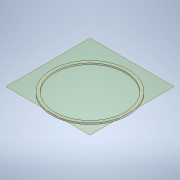
# Autodesk Inventor part: UpperSailCapBottom-ver1-1111-2021
Saved by Autodesk Inventor 2021 (Build 250183000, 183)
## iProperties
Created: 2021-01-28
Part Number: UpperSailCapBottom-ver1-1111-2021
Material: Generic
Document SubType Name: Modeling
Designer: con_c_000
Density: 1 g/cm^3
Appearance: Default
Author: con_c_000
Autodesk Inventor part; units mm, degrees
sketch "Sketch1" plane through (0, 0, 0) normal (0, 1, 0) x (-1, 0, 0)
  circle A0 centre (0, 0) radius 152.4
  circle A1 centre (0, 0) radius 165.1
  dimension "d0" = 304.8
  dimension "d1" = 330.2
  constraints: 2 centre point, 2 coincident
  measures "d0" diameter of A0
  measures "d1" diameter of A1
extrude "Extrusion1" add sketch "Sketch1" along normal blind 152.4
sketch "Sketch2" plane through (0, 0, 0) normal (1, 0, 0) x (0, 1, 0)
  circle A0 centre (100.6077, 0) radius 25.4
  point P0 (0, 0)
  dimension "d4" = 50.8
  constraints: 1 centre point
  measures "d4" diameter of A0
extrude "Extrusion2" add sketch "Sketch2" along normal mid plane 889
sketch "Sketch4" plane through (0, 152.4, 0) normal (0, 1, 0) x (1, 0, 0)
  circle A0 centre (0, 0) radius 152.4
  constraints: 1 centre point, 1 coincident
extrude "Extrusion4" cut sketch "Sketch4" against normal through all
sketch "Sketch5" plane through (0, 152.4, 0) normal (0, 1, 0) x (1, 0, 0)
  circle A0 centre (0, 0) radius 165.1
  constraints: 1 centre point, 1 coincident
extrude "Extrusion5" add sketch "Sketch5" along normal blind 50.8 draft -50
ref_plane "Work Plane2" through (75.376, -18.8821, -44.9646) normal (1, 0, 0) x (0, 1, 0)
ref_plane "Work Plane5" through (0, 25.4, 165.1) normal (0, 0, 1) x (1, 0, 0)
sketch "Sketch11" plane through (0, 25.4, 165.1) normal (0, 0, 1) x (1, 0, 0)
  circle A0 centre (0, 75.2094) radius 25.4
  line L0 (165.1, -25.4) -> (-165.1, -25.4) projected
  point P0 (0, -25.4)
  dimension "d31" = 50.8
  dimension "d32" = 100.6094
  constraints: 1 centre point
  measures "d31" diameter of A0
  measures "d32" distance from line of L0 A0.centre
extrude "Extrusion11" add sketch "Sketch11" along normal blind 280.543
ref_plane "Work Plane6" through (0, 25.4, -165.1) normal (0, 0, 1) x (1, 0, 0)
sketch "Sketch12" plane through (0, 25.4, -165.1) normal (0, 0, 1) x (1, 0, 0)
  circle A0 centre (0, 75.2094) radius 25.4
  line L0 (165.1, -25.4) -> (-165.1, -25.4) projected
  point P0 (0, -25.4)
  dimension "d36" = 50.8
  dimension "d37" = 100.6094
  constraints: 1 centre point
  measures "d36" diameter of A0
  measures "d37" distance from line of L0 A0.centre
extrude "Extrusion12" add sketch "Sketch12" against normal blind 280.543
ref_plane "Work Plane10" through (0, 152.4, 0) normal (0, -1, 0) x (1, 0, 0)
ref_plane "Work Plane9" through (0, 63.5, 0) normal (0, -1, 0) x (1, 0, 0)
sketch "Sketch13" plane through (0, 152.4, 0) normal (0, -1, 0) x (1, 0, 0)
  line L0 (-199.2875, -201.2037) -> (234.7376, -201.2037)
  line L1 (234.7376, -201.2037) -> (234.7376, 210.7848)
  line L2 (234.7376, 210.7848) -> (-199.2875, 210.7848)
  line L3 (-199.2875, 210.7848) -> (-199.2875, -201.2037)
  point P0 (0, 0)
  constraints: 8 end point, 2 parallel, 1 horizontal, 1 perpendicular
extrude "Extrusion13" cut sketch "Sketch13" against normal blind 127
ref_plane "Work Plane11" through (0, 63.5, 0) normal (0, -1, 0) x (1, 0, 0)
sketch "Sketch15" plane through (0, 63.5, 0) normal (0, -1, 0) x (1, 0, 0)
  line L0 (-509.2014, 528.9036) -> (494.7202, 528.9036)
  line L1 (494.7202, 528.9036) -> (494.7202, -498.4488)
  line L2 (494.7202, -498.4488) -> (-509.2014, -498.4488)
  line L3 (-509.2014, -498.4488) -> (-509.2014, 528.9036)
  point P0 (0, 0)
  constraints: 8 end point, 2 parallel, 1 horizontal, 1 perpendicular
extrude "Extrusion15" cut sketch "Sketch15" against normal blind 254
ref_plane "Work Plane12" through (0, 25.4, 0) normal (0, -1, 0) x (1, 0, 0)
sketch "Sketch16" plane through (0, 25.4, 0) normal (0, -1, 0) x (1, 0, 0)
  line L0 (-189.4244, 211.7722) -> (231.9916, 211.7722)
  line L1 (231.9916, 211.7722) -> (231.9916, -229.8633)
  line L2 (231.9916, -229.8633) -> (-189.4244, -229.8633)
  line L3 (-189.4244, -229.8633) -> (-189.4244, 211.7722)
  point P0 (0, 0)
  constraints: 8 end point, 2 parallel, 1 horizontal, 1 perpendicular
extrude "Extrusion16" cut sketch "Sketch16" against normal blind 254
ref_plane "Work Plane14" through (-0.824, -18.8821, -44.9646) normal (1, 0, 0) x (0, 1, 0)
ref_plane "Work Plane13" through (164.276, -18.8821, -44.9646) normal (1, 0, 0) x (0, 1, 0)
ref_plane "Work Plane15" through (0, 25.4, 0) normal (0, -1, 0) x (1, 0, 0)
sketch "Sketch17" plane through (0, 25.4, 0) normal (0, -1, 0) x (1, 0, 0)
  line L0 (-206.305, -203.3787) -> (218.0102, -203.3787)
  line L1 (218.0102, -203.3787) -> (218.0102, 226.7892)
  line L2 (218.0102, 226.7892) -> (-206.305, 226.7892)
  line L3 (-206.305, 226.7892) -> (-206.305, -203.3787)
  point P0 (0, 0)
  constraints: 8 end point, 2 parallel, 1 horizontal, 1 perpendicular
extrude "Extrusion17" cut sketch "Sketch17" along normal blind 19.05
ref_plane "Work Plane8" through (0, 0, 0) normal (0, -1, 0) x (1, 0, 0)
body "Solid1"
